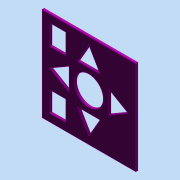
# Autodesk Inventor part: Mat_Tren_Button
Saved by Autodesk Inventor 2016 (Build 200138000, 138)
## iProperties
Created: 2016-08-17
Part Number: Mat_Tren_Button
Material: Rubber
Document SubType Name: Modeling
Designer: ADMIN
Density: 0.93 g/cm^3
Appearance: Smooth - Purple
Author: ADMIN
Autodesk Inventor part; units mm, degrees
ref_plane "YZ Plane" through (0, 0, 0) normal (1, 0, 0) x (0, 1, 0)
ref_plane "XZ Plane" through (0, 0, 0) normal (0, 1, 0) x (-1, 0, 0)
ref_plane "XY Plane" through (0, 0, 0) normal (0, 0, 1) x (1, 0, 0)
sketch "Sketch1" plane through (0, 0, 0) normal (0, 1, 0) x (-1, 0, 0)
  circle A0 centre (0, 0) radius 15
  line L0 (0, -25) -> (10, -25)
  line L1 (0, -25) -> (-10, -25)
  line L2 (-10, -25) -> (0, -42.3205)
  line L3 (0, -42.3205) -> (10, -25)
  circle A1 centre (0, 0) radius 16.5
  line L4 (12.5981, -23.5) -> (0.866, -23.5)
  line L5 (0.866, -23.5) -> (-12.5981, -23.5)
  line L6 (-12.5981, -23.5) -> (0, -45.3205)
  line L7 (0, -45.3205) -> (12.5981, -23.5)
  line L8 (25, 0) -> (25, 10)
  line L9 (25, 0) -> (25, -10)
  line L10 (25, -10) -> (42.3205, 0)
  line L11 (42.3205, 0) -> (25, 10)
  line L12 (23.5, 12.5981) -> (23.5, 0.866)
  line L13 (23.5, 0.866) -> (23.5, -12.5981)
  line L14 (23.5, -12.5981) -> (45.3205, 0)
  line L15 (45.3205, 0) -> (23.5, 12.5981)
  line L16 (0, 25) -> (-10, 25)
  line L17 (0, 25) -> (10, 25)
  line L18 (10, 25) -> (0, 42.3205)
  line L19 (0, 42.3205) -> (-10, 25)
  line L20 (-12.5981, 23.5) -> (-0.866, 23.5)
  line L21 (-0.866, 23.5) -> (12.5981, 23.5)
  line L22 (12.5981, 23.5) -> (0, 45.3205)
  line L23 (0, 45.3205) -> (-12.5981, 23.5)
  line L24 (-25, 0) -> (-25, -10)
  line L25 (-25, 0) -> (-25, 10)
  line L26 (-25, 10) -> (-42.3205, 0)
  line L27 (-42.3205, 0) -> (-25, -10)
  line L28 (-23.5, -12.5981) -> (-23.5, -0.866)
  line L29 (-23.5, -0.866) -> (-23.5, 12.5981)
  line L30 (-23.5, 12.5981) -> (-45.3205, 0)
  line L31 (-45.3205, 0) -> (-23.5, -12.5981)
  line L32 (45.3205, 45.3205) -> (27.3205, 45.3205)
  line L33 (27.3205, 45.3205) -> (27.3205, 22.3205)
  line L34 (27.3205, 22.3205) -> (45.3205, 22.3205)
  line L35 (45.3205, 22.3205) -> (45.3205, 45.3205)
  line L36 (28.8205, 23.8205) -> (28.8205, 43.8205)
  line L37 (28.8205, 43.8205) -> (43.8205, 43.8205)
  line L38 (43.8205, 43.8205) -> (43.8205, 23.8205)
  line L39 (43.8205, 23.8205) -> (28.8205, 23.8205)
  line L40 (45.3205, -45.3205) -> (27.3205, -45.3205)
  line L41 (27.3205, -45.3205) -> (27.3205, -22.3205)
  line L42 (27.3205, -22.3205) -> (45.3205, -22.3205)
  line L43 (45.3205, -22.3205) -> (45.3205, -45.3205)
  line L44 (28.8205, -23.8205) -> (28.8205, -43.8205)
  line L45 (28.8205, -43.8205) -> (43.8205, -43.8205)
  line L46 (43.8205, -43.8205) -> (43.8205, -23.8205)
  line L47 (43.8205, -23.8205) -> (28.8205, -23.8205)
  line L48 (0, 55) -> (55, 55)
  line L49 (55, 55) -> (55, -55)
  line L50 (55, -55) -> (-55, -55)
  line L51 (-55, -55) -> (-55, 55)
  line L52 (-55, 55) -> (0, 55)
  dimension "d1" = 10
  dimension "d2" = 10
  dimension "d3" = 20
  dimension "d4" = 60
  dimension "d6" = 1.5
  dimension "d7" = 25
  dimension "d10" = 360
  dimension "d12" = 18
  dimension "d13" = 23
  dimension "d14" = 1.5
  dimension "d16" = 55
  dimension "d17" = 110
  dimension "d18" = 110
  dimension "d19" = 110
  constraints: 106 end point, 4 horizontal, 4 parallel, 4 perpendicular, 2 centre point, 2 coincident, 1 point on line, 71 other
  measures "d1" distance of L0.start L0.end
  measures "d2" distance of L0.start L1.end
  measures "d3" distance of L1.end L2.end
  measures "d4" angle of L2 L1
  measures "d6" distance between parallel lines of L0 L4
  measures "d7" distance of point (0, 0) L0.start
  measures "d12" distance of L34.end L33.end
  measures "d13" distance of L33.end L32.end
  measures "d14" distance between parallel lines of L33 L36
  measures "d16" distance of L48.start L48.end
  measures "d17" distance of L48.end L49.end
  measures "d18" distance of L49.end L50.end
  measures "d19" distance of L50.end L51.end
extrude "Extrusion1" add sketch "Sketch1" along normal blind 3 contours L48 L49 L50 L51 L52
fillet "Fillet1" radius 0.5 12 edges at (0, 3, -55) (55, 3, 0) (-55, 3, 0) (27.5, 3, 55) (-55, 0, 0) (0, 0, -55) (-55, 1.5, -55) (-55, 1.5, 55) (-27.5, 0, 55) (55, 1.5, 55) (55, 0, 0) (55, 1.5, -55)
fillet "Fillet2" radius 0.5 42 edges at (16.5, 3, 0) (16.5, 0, 0) (6.299, 3, -34.4103) (5.866, 3, -23.5) (-6.299, 3, -34.4103) (-27.3205, 3, -33.8205) (-36.3205, 3, -45.3205) (-45.3205, 3, -33.8205) (-36.3205, 3, -22.3205) (-34.4103, 3, -6.299) (-34.4103, 3, 6.299) (-23.5, 3, -5.866) (-36.3205, 3, 22.3205) (-27.3205, 3, 33.8205) (-45.3205, 3, 33.8205) (-36.3205, 3, 45.3205) (-6.299, 3, 34.4103) (6.299, 3, 34.4103) (-5.866, 3, 23.5) (34.4103, 3, 6.299) (34.4103, 3, -6.299) (23.5, 3, 5.866) (-36.3205, 0, 45.3205) (-45.3205, 0, 33.8205) (-36.3205, 0, 22.3205) (-27.3205, 0, 33.8205) (-5.866, 0, 23.5) (6.299, 0, 34.4103) (-6.299, 0, 34.4103) (-34.4103, 0, -6.299) (-34.4103, 0, 6.299) (-23.5, 0, -5.866) (-45.3205, 0, -33.8205) (-36.3205, 0, -22.3205) (-27.3205, 0, -33.8205) (-36.3205, 0, -45.3205) (-6.299, 0, -34.4103) (5.866, 0, -23.5) (6.299, 0, -34.4103) (23.5, 0, 5.866) (34.4103, 0, -6.299) (34.4103, 0, 6.299)
body "Solid1"
